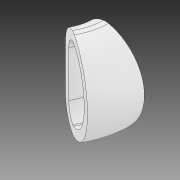
# Autodesk Inventor part: L_20uH-Wedge
Saved by Autodesk Inventor 2021 (Build 250183000, 183)
## iProperties
Created: 2020-11-13
Part Number: L_20uH-Wedge
Material: UHMW, White
Document SubType Name: Modeling
Designer: Eli Mattingly
Density: 0.94 g/cm^3
Appearance: Smooth - White
Author: Eli Mattingly
Autodesk Inventor part; units mm, degrees
ref_plane "Work Plane2" through (0, 0, 0) normal (-0.2588, 0, -0.9659) x (0, 1, 0)
ref_plane "Work Plane1" through (-7, 0, -29.5697) normal (1, 0, 0) x (0, 0, -1)
ref_plane "YZ Plane" through (0, 0, 0) normal (1, 0, 0) x (0, 1, 0)
sketch "Sketch1" plane through (0, 0, 0) normal (0, 0, 1) x (1, 0, 0)
  line L0 (0, 0) -> (0, 15.36) construction
  line L1 (10.24, 7.86) -> (10.24, -7.86)
  line L2 (17.74, 15.36) -> (17.74, -15.36) construction
  arc A0 (16.6996, 15.2875) -> (10.24, 7.86) centre (17.74, 7.86) ccw
  arc A1 (10.24, -7.86) -> (16.6996, -15.2875) centre (17.74, -7.86) ccw
  arc A2 (18.4574, -15.2213) -> (18.4574, 15.2213) centre (15.1418, 0) ccw
  line L3 (0, 0) -> (51.4073, 0)
  arc A3 (18.4574, 15.2213) -> (16.6996, 15.2875) centre (17.3932, 10.3358) ccw
  arc A4 (16.6996, -15.2875) -> (18.4574, -15.2213) centre (17.3932, -10.3358) ccw
  arc A5 (17.8189, 12.29) -> (17.1158, 12.3165) centre (17.3932, 10.3358) ccw
  arc A6 (17.1158, 12.3165) -> (13.24, 7.86) centre (17.74, 7.86) ccw
  line L4 (13.24, 7.86) -> (13.24, -7.86)
  arc A7 (13.24, -7.86) -> (17.1158, -12.3165) centre (17.74, -7.86) ccw
  arc A8 (17.1158, -12.3165) -> (17.8189, -12.29) centre (17.3932, -10.3358) ccw
  arc A9 (17.8189, -12.29) -> (17.8189, 12.29) centre (15.1418, 0) ccw
  point P0 (10.24, 0)
  point P1 (30.72, 0)
  point P2 (17.74, 0)
  dimension "MaxHeight" = 15.36
  dimension "FlatHeightx2" = 15.72
  dimension "ID" = 20.48
  dimension "OD" = 61.44
  dimension "d5" = 30.72
  dimension "RadAtPeak" = 17.74
  dimension "d90" = 5
  dimension "d97" = 3
  constraints: 25 point on circle, 10 centre point, 10 end point, 5 tangent, 3 horizontal alignment, 3 vertical, 2 line through centre, 2 midpoint, 1 equal radius, 1 horizontal, 5 other
  measures "MaxHeight" distance of L0.start L0.end
  measures "FlatHeightx2" distance of L1.start L1.end
  measures "ID" diameter of L1 L0
  measures "OD" diameter of point (30.72, 0) L0
  measures "d5" distance of L2.start L2.end
  measures "RadAtPeak" distance from line of L0.start L2
  measures "d90" radius of A3
  measures "d97" radial gap between concentric circles of A2 A9
revolve "Revolution1" add sketch "Sketch1" angle 30 about axis through (0, 0, 0) along (0, -1, 0) contours A0 A3 A2 L3 A9 A5 A6 L4 L1 | L3 L4 A7 A8 A9 A2 A4 A1 L1
sketch "Sketch7" plane through (0, 0, 0) normal (0, 1, 0) x (-1, 0, 0)
  circle A0 centre (0, 0) radius 198.9616
  constraints: 1 centre point, 1 coincident
sketch "Sketch8" plane through (0, 0, 0) normal (1, 0, 0) x (0, 1, 0)
  circle A0 centre (0, 0) radius 159.0195
  constraints: 1 centre point, 1 coincident
sketch "Sketch9" plane through (0, 0, 0) normal (1, 0, 0) x (0, 0, -1)
  line L0 (74, 0) -> (35, 0) projected
  point P0 (0, 0)
  point P1 (-52.5, 0)
  point P2 (0, 0)
  point P3 (52.5, 0)
  dimension "d88" = 105
  dimension "d89" = 52.5
  constraints: 1 point on line
  measures "d88" distance of point (52.5, 0) point (-52.5, 0)
  measures "d89" distance of point (52.5, 0) point (0, 0)
sketch "Sketch11" plane through (0, 0, 0) normal (1, 0, 0) x (0, 0, -1)
  arc A0 (-35, 25.9107) -> (-42.6927, 34.8921) centre (-44.0893, 25.9107) ccw projected
  line L0 (-35, 25.9107) -> (-35, 0) projected
  line L1 (-35, 0) -> (35, 0) projected
  arc A1 (-50.0415, 0) -> (-54.9585, 0) centre (-52.5, 0) ccw projected
  arc A2 (-50.0415, 0) -> (-54.9585, 0) centre (-37.5, 0) ccw projected
  arc A3 (-39.8678, 39.0634) -> (-73, 0) centre (-33.4058, 0) ccw
  arc A4 (-29.5697, 27.789) -> (-36.4391, 38.3935) centre (-44.0893, 25.9107) ccw
  line L2 (-29.5697, 27.789) -> (-29.5697, 0)
  line L3 (-35, 0) -> (35, 0) projected
  line L4 (-73, 0) -> (-29.5697, 0)
  arc A5 (-36.4391, 38.3935) -> (-39.8678, 39.0634) centre (-39.0518, 34.1304) ccw
  point P0 (0, 0)
  point P1 (-35, 0)
  point P2 (-29.5697, 0)
  point P3 (-54.9585, 0)
  point P4 (-50.0415, 0)
  dimension "d91" = 5
  constraints: 6 point on circle, 4 end point, 3 centre point, 2 tangent, 1 horizontal, 1 point on line, 1 other
  measures "d91" radius of A5
equation "\"d5\" = 2 * MaxHeight"
equation "\"d63_Copy\" = 35"
body "Solid1"
